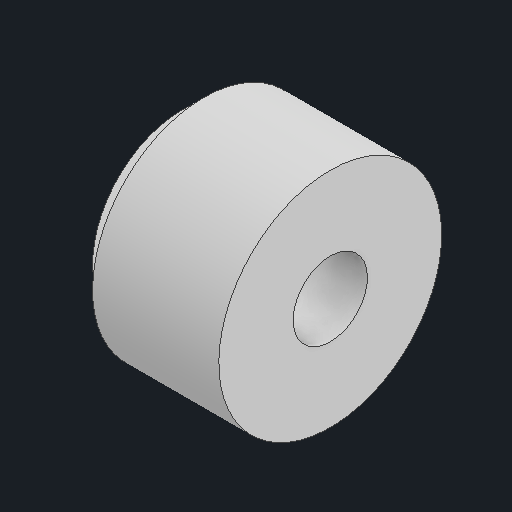
# Autodesk Inventor part: a_full_angledim
Saved by Autodesk Inventor 2027 (Build 310192060, 192F)
## iProperties
Created: 2026-07-13
Part Number: a_full_angledim
Material: Generic
Document SubType Name: Modeling
Designer: vmiguel
Density: 1 g/cm^3
Appearance: Default
Author: vmiguel
Autodesk Inventor part; units mm, degrees
ref_plane "YZ Plane" through (0, 0, 0) normal (1, 0, 0) x (0, 1, 0)
ref_plane "XZ Plane" through (0, 0, 0) normal (0, 1, 0) x (-1, 0, 0)
ref_plane "XY Plane" through (0, 0, 0) normal (0, 0, 1) x (1, 0, 0)
sketch "Sketch1" plane through (0, 0, 0) normal (0, 0, 1) x (1, 0, 0)
  line L0 (10, 5) -> (30, 5)
  line L1 (30, 5) -> (30, 15)
  line L2 (30, 15) -> (13, 15)
  line L3 (13, 15) -> (10, 12)
  line L4 (10, 12) -> (10, 5)
  line L5 (6, 0) -> (34, 0) projected
  dimension "d0" = 135
  constraints: 10 end point
  measures "d0" angle of L3 L4
revolve "Revolution1" add sketch "Sketch1" angle 360 about axis through (-10, 0, 0) along (1, 0, 0)
body "Solid1"
